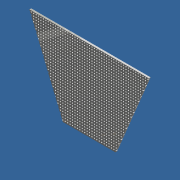
# Autodesk Inventor part: Detektorplatine
Saved by Autodesk Inventor 2018 (Build 220112000, 112)
## iProperties
Created: 2018-11-01
Part Number: Detektorplatine
Material: PC/ABS-Kunststoff
Document SubType Name: Modeling
Designer: M.Knabel
Density: 0.357273 g/cm^3
Appearance: Glatt - weiß
Mass: 2.14367 g
Surface Area: 141.537 cm^2
Volume: 6.0001 cm^3
Author: M.Knabel
Autodesk Inventor part; units mm, degrees
ref_plane "YZ Plane" through (0, 0, 0) normal (1, 0, 0) x (0, 1, 0)
ref_plane "XZ Plane" through (0, 0, 0) normal (0, 1, 0) x (-1, 0, 0)
ref_plane "XY Plane" through (0, 0, 0) normal (0, 0, 1) x (1, 0, 0)
sketch "Skizze1" plane through (0, 0, 0) normal (0, 1, 0) x (-1, 0, 0)
  line L0 (-50.2277, 69) -> (50.2277, 69)
  line L1 (50.2277, 69) -> (21.647, 0)
  line L2 (21.647, 0) -> (-21.647, 0)
  line L3 (-21.647, 0) -> (-50.2277, 69)
  line L4 (0, -13.8) -> (0, 82.8) construction
  line L5 (70.3188, 0) -> (-70.3188, 0) construction
  point P0 (0, 0)
  dimension "d0" = 43.294
  dimension "d1" = 112.5
  dimension "d2" = 69
  constraints: 8 end point, 1 collinear, 1 horizontal, 1 parallel, 1 other
  measures "d0" distance of L1.end L2.end
  measures "d1" angle of L2 L3
  measures "d2" distance between parallel lines of L2 L0
extrude "Extrusion1" add sketch "Skizze1" along normal blind 1.5
sketch "Skizze2" plane through (0, 1.5, 0) normal (0, 1, 0) x (1, 0, 0)
  line L0 (21.647, 0) -> (-21.647, 0) projected
  line L1 (-21.647, 0) -> (-21.647, 7.3765) construction
  point P0 (0, 0)
  point P1 (-21.647, -1.5)
  point P2 (-19.647, -1.5)
  point P3 (-17.647, -1.5)
  point P4 (-15.647, -1.5)
  point P5 (-13.647, -1.5)
  point P6 (-11.647, -1.5)
  point P7 (-9.647, -1.5)
  point P8 (-7.647, -1.5)
  point P9 (-5.647, -1.5)
  point P10 (-3.647, -1.5)
  point P11 (-1.647, -1.5)
  point P12 (0.353, -1.5)
  point P13 (2.353, -1.5)
  point P14 (4.353, -1.5)
  point P15 (6.353, -1.5)
  point P16 (8.353, -1.5)
  point P17 (10.353, -1.5)
  point P18 (12.353, -1.5)
  point P19 (14.353, -1.5)
  point P20 (16.353, -1.5)
  point P21 (18.353, -1.5)
  point P22 (20.353, -1.5)
  point P23 (22.353, -1.5)
  point P24 (22.353, -3.5)
  point P25 (20.353, -3.5)
  point P26 (18.353, -3.5)
  point P27 (16.353, -3.5)
  point P28 (14.353, -3.5)
  point P29 (12.353, -3.5)
  point P30 (10.353, -3.5)
  point P31 (8.353, -3.5)
  point P32 (6.353, -3.5)
  point P33 (4.353, -3.5)
  point P34 (2.353, -3.5)
  point P35 (0.353, -3.5)
  point P36 (-1.647, -3.5)
  point P37 (-3.647, -3.5)
  point P38 (-5.647, -3.5)
  point P39 (-7.647, -3.5)
  point P40 (-9.647, -3.5)
  point P41 (-11.647, -3.5)
  point P42 (-13.647, -3.5)
  point P43 (-15.647, -3.5)
  point P44 (-17.647, -3.5)
  point P45 (-19.647, -3.5)
  point P46 (-21.647, -3.5)
  point P47 (22.353, -5.5)
  point P48 (20.353, -5.5)
  point P49 (18.353, -5.5)
  point P50 (16.353, -5.5)
  point P51 (14.353, -5.5)
  point P52 (12.353, -5.5)
  point P53 (10.353, -5.5)
  point P54 (8.353, -5.5)
  point P55 (6.353, -5.5)
  point P56 (4.353, -5.5)
  point P57 (2.353, -5.5)
  point P58 (0.353, -5.5)
  point P59 (-1.647, -5.5)
  point P60 (-3.647, -5.5)
  point P61 (-5.647, -5.5)
  point P62 (-7.647, -5.5)
  point P63 (-9.647, -5.5)
  point P64 (-11.647, -5.5)
  point P65 (-13.647, -5.5)
  point P66 (-15.647, -5.5)
  point P67 (-17.647, -5.5)
  point P68 (-19.647, -5.5)
  point P69 (-21.647, -5.5)
  point P70 (22.353, -7.5)
  point P71 (20.353, -7.5)
  point P72 (18.353, -7.5)
  point P73 (16.353, -7.5)
  point P74 (14.353, -7.5)
  point P75 (12.353, -7.5)
  point P76 (10.353, -7.5)
  point P77 (8.353, -7.5)
  point P78 (6.353, -7.5)
  point P79 (4.353, -7.5)
  point P80 (2.353, -7.5)
  point P81 (0.353, -7.5)
  point P82 (-1.647, -7.5)
  point P83 (-3.647, -7.5)
  point P84 (-5.647, -7.5)
  point P85 (-7.647, -7.5)
  point P86 (-9.647, -7.5)
  point P87 (-11.647, -7.5)
  point P88 (-13.647, -7.5)
  point P89 (-15.647, -7.5)
  point P90 (-17.647, -7.5)
  point P91 (-19.647, -7.5)
  point P92 (-21.647, -7.5)
  point P93 (22.353, -9.5)
  point P94 (20.353, -9.5)
  point P95 (18.353, -9.5)
  point P96 (16.353, -9.5)
  point P97 (14.353, -9.5)
  point P98 (12.353, -9.5)
  point P99 (10.353, -9.5)
  point P100 (8.353, -9.5)
  point P101 (6.353, -9.5)
  point P102 (4.353, -9.5)
  point P103 (2.353, -9.5)
  point P104 (0.353, -9.5)
  point P105 (-1.647, -9.5)
  point P106 (-3.647, -9.5)
  point P107 (-5.647, -9.5)
  point P108 (-7.647, -9.5)
  point P109 (-9.647, -9.5)
  point P110 (-11.647, -9.5)
  point P111 (-13.647, -9.5)
  point P112 (-15.647, -9.5)
  point P113 (-17.647, -9.5)
  point P114 (-19.647, -9.5)
  point P115 (-21.647, -9.5)
  point P116 (22.353, -11.5)
  point P117 (20.353, -11.5)
  point P118 (18.353, -11.5)
  point P119 (16.353, -11.5)
  point P120 (14.353, -11.5)
  point P121 (12.353, -11.5)
  point P122 (10.353, -11.5)
  point P123 (8.353, -11.5)
  point P124 (6.353, -11.5)
  point P125 (4.353, -11.5)
  point P126 (2.353, -11.5)
  point P127 (0.353, -11.5)
  point P128 (-1.647, -11.5)
  point P129 (-3.647, -11.5)
  point P130 (-5.647, -11.5)
  point P131 (-7.647, -11.5)
  point P132 (-9.647, -11.5)
  point P133 (-11.647, -11.5)
  point P134 (-13.647, -11.5)
  point P135 (-15.647, -11.5)
  point P136 (-17.647, -11.5)
  point P137 (-19.647, -11.5)
  point P138 (-21.647, -11.5)
  point P139 (22.353, -13.5)
  point P140 (20.353, -13.5)
  point P141 (18.353, -13.5)
  point P142 (16.353, -13.5)
  point P143 (14.353, -13.5)
  point P144 (12.353, -13.5)
  point P145 (10.353, -13.5)
  point P146 (8.353, -13.5)
  point P147 (6.353, -13.5)
  point P148 (4.353, -13.5)
  point P149 (2.353, -13.5)
  point P150 (0.353, -13.5)
  point P151 (-1.647, -13.5)
  point P152 (-3.647, -13.5)
  point P153 (-5.647, -13.5)
  point P154 (-7.647, -13.5)
  point P155 (-9.647, -13.5)
  point P156 (-11.647, -13.5)
  point P157 (-13.647, -13.5)
  point P158 (-15.647, -13.5)
  point P159 (-17.647, -13.5)
  point P160 (-19.647, -13.5)
  point P161 (-21.647, -13.5)
  point P162 (22.353, -15.5)
  point P163 (20.353, -15.5)
  point P164 (18.353, -15.5)
  point P165 (16.353, -15.5)
  point P166 (14.353, -15.5)
  point P167 (12.353, -15.5)
  point P168 (10.353, -15.5)
  point P169 (8.353, -15.5)
  point P170 (6.353, -15.5)
  point P171 (4.353, -15.5)
  point P172 (2.353, -15.5)
  point P173 (0.353, -15.5)
  point P174 (-1.647, -15.5)
  point P175 (-3.647, -15.5)
  point P176 (-5.647, -15.5)
  point P177 (-7.647, -15.5)
  point P178 (-9.647, -15.5)
  point P179 (-11.647, -15.5)
  point P180 (-13.647, -15.5)
  point P181 (-15.647, -15.5)
  point P182 (-17.647, -15.5)
  point P183 (-19.647, -15.5)
  point P184 (-21.647, -15.5)
  point P185 (22.353, -17.5)
  point P186 (20.353, -17.5)
  point P187 (18.353, -17.5)
  point P188 (16.353, -17.5)
  point P189 (14.353, -17.5)
  point P190 (12.353, -17.5)
  point P191 (10.353, -17.5)
  point P192 (8.353, -17.5)
  point P193 (6.353, -17.5)
  point P194 (4.353, -17.5)
  point P195 (2.353, -17.5)
  point P196 (0.353, -17.5)
  point P197 (-1.647, -17.5)
  point P198 (-3.647, -17.5)
  point P199 (-5.647, -17.5)
  dimension "d5" = 1.5
  dimension "d8" = 2
  dimension "d15" = 2
  dimension "d22" = 2
  dimension "d29" = 2
  constraints: 3 horizontal, 2 end point, 2 vertical, 1 point on line, 1665 other
  measures "d5" distance from line of L0 point (-21.647, -1.5)
  measures "d8" distance of point (-21.647, -1.5) point (-19.647, -1.5)
  measures "d15" distance of point (22.353, -1.5) point (22.353, -3.5)
  measures "d22" distance of point (22.353, -67.5) point (24.353, -67.5)
  measures "d29" distance of point (-21.647, -67.5) point (-23.647, -67.5)
hole "Bohrung1" at (-21.647, 1.5, 1.5) at (-19.647, 1.5, 1.5) at (-17.647, 1.5, 1.5) at (-15.647, 1.5, 1.5) at (-13.647, 1.5, 1.5) at (-11.647, 1.5, 1.5) at (-9.647, 1.5, 1.5) at (-7.647, 1.5, 1.5) at (-5.647, 1.5, 1.5) at (-3.647, 1.5, 1.5) at (-1.647, 1.5, 1.5) at (0.353, 1.5, 1.5) at (2.353, 1.5, 1.5) at (4.353, 1.5, 1.5) at (6.353, 1.5, 1.5) at (8.353, 1.5, 1.5) at (10.353, 1.5, 1.5) at (12.353, 1.5, 1.5) at (14.353, 1.5, 1.5) at (16.353, 1.5, 1.5) at (18.353, 1.5, 1.5) at (20.353, 1.5, 1.5) at (22.353, 1.5, 1.5) at (22.353, 1.5, 3.5) at (20.353, 1.5, 3.5) at (18.353, 1.5, 3.5) at (16.353, 1.5, 3.5) at (14.353, 1.5, 3.5) at (12.353, 1.5, 3.5) at (10.353, 1.5, 3.5) at (8.353, 1.5, 3.5) at (6.353, 1.5, 3.5) at (4.353, 1.5, 3.5) at (2.353, 1.5, 3.5) at (0.353, 1.5, 3.5) at (-1.647, 1.5, 3.5) at (-3.647, 1.5, 3.5) at (-5.647, 1.5, 3.5) at (-7.647, 1.5, 3.5) at (-9.647, 1.5, 3.5) at (-11.647, 1.5, 3.5) at (-13.647, 1.5, 3.5) at (-15.647, 1.5, 3.5) at (-17.647, 1.5, 3.5) at (-19.647, 1.5, 3.5) at (-21.647, 1.5, 3.5) at (22.353, 1.5, 5.5) at (20.353, 1.5, 5.5) at (18.353, 1.5, 5.5) at (16.353, 1.5, 5.5) direction (0, -1, 0) diameter 1 end through all and at (14.353, 1.5, 5.5) (12.353, 1.5, 5.5) (10.353, 1.5, 5.5) (8.353, 1.5, 5.5) (6.353, 1.5, 5.5) (4.353, 1.5, 5.5) (2.353, 1.5, 5.5) (0.353, 1.5, 5.5) (-1.647, 1.5, 5.5) (-3.647, 1.5, 5.5) (-5.647, 1.5, 5.5) (-7.647, 1.5, 5.5) (-9.647, 1.5, 5.5) (-11.647, 1.5, 5.5) (-13.647, 1.5, 5.5) (-15.647, 1.5, 5.5) (-17.647, 1.5, 5.5) (-19.647, 1.5, 5.5) (-21.647, 1.5, 5.5) (22.353, 1.5, 7.5) (20.353, 1.5, 7.5) (18.353, 1.5, 7.5) (16.353, 1.5, 7.5) (14.353, 1.5, 7.5) (12.353, 1.5, 7.5) (10.353, 1.5, 7.5) (8.353, 1.5, 7.5) (6.353, 1.5, 7.5) (4.353, 1.5, 7.5) (2.353, 1.5, 7.5) (0.353, 1.5, 7.5) (-1.647, 1.5, 7.5) (-3.647, 1.5, 7.5) (-5.647, 1.5, 7.5) (-7.647, 1.5, 7.5) (-9.647, 1.5, 7.5) (-11.647, 1.5, 7.5) (-13.647, 1.5, 7.5) (-15.647, 1.5, 7.5) (-17.647, 1.5, 7.5) (-19.647, 1.5, 7.5) (-21.647, 1.5, 7.5) (22.353, 1.5, 9.5) (20.353, 1.5, 9.5) (18.353, 1.5, 9.5) (16.353, 1.5, 9.5) (14.353, 1.5, 9.5) (12.353, 1.5, 9.5) (10.353, 1.5, 9.5) (8.353, 1.5, 9.5) (6.353, 1.5, 9.5) (4.353, 1.5, 9.5) (2.353, 1.5, 9.5) (0.353, 1.5, 9.5) (-1.647, 1.5, 9.5) (-3.647, 1.5, 9.5) (-5.647, 1.5, 9.5) (-7.647, 1.5, 9.5) (-9.647, 1.5, 9.5) (-11.647, 1.5, 9.5) (-13.647, 1.5, 9.5) (-15.647, 1.5, 9.5) (-17.647, 1.5, 9.5) (-19.647, 1.5, 9.5) (-21.647, 1.5, 9.5) (22.353, 1.5, 11.5) (20.353, 1.5, 11.5) (18.353, 1.5, 11.5) (16.353, 1.5, 11.5) (14.353, 1.5, 11.5) (12.353, 1.5, 11.5) (10.353, 1.5, 11.5) (8.353, 1.5, 11.5) (6.353, 1.5, 11.5) (4.353, 1.5, 11.5) (2.353, 1.5, 11.5) (0.353, 1.5, 11.5) (-1.647, 1.5, 11.5) (-3.647, 1.5, 11.5) (-5.647, 1.5, 11.5) (-7.647, 1.5, 11.5) (-9.647, 1.5, 11.5) (-11.647, 1.5, 11.5) (-13.647, 1.5, 11.5) (-15.647, 1.5, 11.5) (-17.647, 1.5, 11.5) (-19.647, 1.5, 11.5) (-21.647, 1.5, 11.5) (22.353, 1.5, 13.5) (20.353, 1.5, 13.5) (18.353, 1.5, 13.5) (16.353, 1.5, 13.5) (14.353, 1.5, 13.5) (12.353, 1.5, 13.5) (10.353, 1.5, 13.5) (8.353, 1.5, 13.5) (6.353, 1.5, 13.5) (4.353, 1.5, 13.5) (2.353, 1.5, 13.5) (0.353, 1.5, 13.5) (-1.647, 1.5, 13.5) (-3.647, 1.5, 13.5) (-5.647, 1.5, 13.5) (-7.647, 1.5, 13.5) (-9.647, 1.5, 13.5) (-11.647, 1.5, 13.5) (-13.647, 1.5, 13.5) (-15.647, 1.5, 13.5) (-17.647, 1.5, 13.5) (-19.647, 1.5, 13.5) (-21.647, 1.5, 13.5) (22.353, 1.5, 15.5) (20.353, 1.5, 15.5) (18.353, 1.5, 15.5) (16.353, 1.5, 15.5) (14.353, 1.5, 15.5) (12.353, 1.5, 15.5) (10.353, 1.5, 15.5) (8.353, 1.5, 15.5) (6.353, 1.5, 15.5) (4.353, 1.5, 15.5) (2.353, 1.5, 15.5) (0.353, 1.5, 15.5) (-1.647, 1.5, 15.5) (-3.647, 1.5, 15.5) (-5.647, 1.5, 15.5) (-7.647, 1.5, 15.5) (-9.647, 1.5, 15.5) (-11.647, 1.5, 15.5) (-13.647, 1.5, 15.5) (-15.647, 1.5, 15.5) (-17.647, 1.5, 15.5) (-19.647, 1.5, 15.5) (-21.647, 1.5, 15.5) (22.353, 1.5, 17.5) (20.353, 1.5, 17.5) (18.353, 1.5, 17.5) (16.353, 1.5, 17.5) (14.353, 1.5, 17.5) (12.353, 1.5, 17.5) (10.353, 1.5, 17.5) (8.353, 1.5, 17.5) (6.353, 1.5, 17.5) (4.353, 1.5, 17.5) (2.353, 1.5, 17.5) (0.353, 1.5, 17.5) (-1.647, 1.5, 17.5) (-3.647, 1.5, 17.5) (-5.647, 1.5, 17.5) (-7.647, 1.5, 17.5) (-9.647, 1.5, 17.5) (-11.647, 1.5, 17.5) (-13.647, 1.5, 17.5) (-15.647, 1.5, 17.5) (-17.647, 1.5, 17.5) (-19.647, 1.5, 17.5) (-21.647, 1.5, 17.5) (22.353, 1.5, 19.5) (20.353, 1.5, 19.5) (18.353, 1.5, 19.5) (16.353, 1.5, 19.5) (14.353, 1.5, 19.5) (12.353, 1.5, 19.5) (10.353, 1.5, 19.5) (8.353, 1.5, 19.5) (6.353, 1.5, 19.5) (4.353, 1.5, 19.5) (2.353, 1.5, 19.5) (0.353, 1.5, 19.5) (-1.647, 1.5, 19.5) (-3.647, 1.5, 19.5) (-5.647, 1.5, 19.5) (-7.647, 1.5, 19.5) (-9.647, 1.5, 19.5) (-11.647, 1.5, 19.5) (-13.647, 1.5, 19.5) (-15.647, 1.5, 19.5) (-17.647, 1.5, 19.5) (-19.647, 1.5, 19.5) (-21.647, 1.5, 19.5) (22.353, 1.5, 21.5) (20.353, 1.5, 21.5) (18.353, 1.5, 21.5) (16.353, 1.5, 21.5) (14.353, 1.5, 21.5) (12.353, 1.5, 21.5) (10.353, 1.5, 21.5) (8.353, 1.5, 21.5) (6.353, 1.5, 21.5) (4.353, 1.5, 21.5) (2.353, 1.5, 21.5) (0.353, 1.5, 21.5) (-1.647, 1.5, 21.5) (-3.647, 1.5, 21.5) (-5.647, 1.5, 21.5) (-7.647, 1.5, 21.5) (-9.647, 1.5, 21.5) (-11.647, 1.5, 21.5) (-13.647, 1.5, 21.5) (-15.647, 1.5, 21.5) (-17.647, 1.5, 21.5) (-19.647, 1.5, 21.5) (-21.647, 1.5, 21.5) (22.353, 1.5, 23.5) (20.353, 1.5, 23.5) (18.353, 1.5, 23.5) (16.353, 1.5, 23.5) (14.353, 1.5, 23.5) (12.353, 1.5, 23.5) (10.353, 1.5, 23.5) (8.353, 1.5, 23.5) (6.353, 1.5, 23.5) (4.353, 1.5, 23.5) (2.353, 1.5, 23.5) (0.353, 1.5, 23.5) (-1.647, 1.5, 23.5) (-3.647, 1.5, 23.5) (-5.647, 1.5, 23.5) (-7.647, 1.5, 23.5) (-9.647, 1.5, 23.5) (-11.647, 1.5, 23.5) (-13.647, 1.5, 23.5) (-15.647, 1.5, 23.5) (-17.647, 1.5, 23.5) (-19.647, 1.5, 23.5) (-21.647, 1.5, 23.5) (22.353, 1.5, 25.5) (20.353, 1.5, 25.5) (18.353, 1.5, 25.5) (16.353, 1.5, 25.5) (14.353, 1.5, 25.5) (12.353, 1.5, 25.5) (10.353, 1.5, 25.5) (8.353, 1.5, 25.5) (6.353, 1.5, 25.5) (4.353, 1.5, 25.5) (2.353, 1.5, 25.5) (0.353, 1.5, 25.5) (-1.647, 1.5, 25.5) (-3.647, 1.5, 25.5) (-5.647, 1.5, 25.5) (-7.647, 1.5, 25.5) (-9.647, 1.5, 25.5) (-11.647, 1.5, 25.5) (-13.647, 1.5, 25.5) (-15.647, 1.5, 25.5) (-17.647, 1.5, 25.5) (-19.647, 1.5, 25.5) (-21.647, 1.5, 25.5) (22.353, 1.5, 27.5) (20.353, 1.5, 27.5) (18.353, 1.5, 27.5) (16.353, 1.5, 27.5) (14.353, 1.5, 27.5) (12.353, 1.5, 27.5) (10.353, 1.5, 27.5) (8.353, 1.5, 27.5) (6.353, 1.5, 27.5) (4.353, 1.5, 27.5) (2.353, 1.5, 27.5) (0.353, 1.5, 27.5) (-1.647, 1.5, 27.5) (-3.647, 1.5, 27.5) (-5.647, 1.5, 27.5) (-7.647, 1.5, 27.5) (-9.647, 1.5, 27.5) (-11.647, 1.5, 27.5) (-13.647, 1.5, 27.5) (-15.647, 1.5, 27.5) (-17.647, 1.5, 27.5) (-19.647, 1.5, 27.5) (-21.647, 1.5, 27.5) (22.353, 1.5, 29.5) (20.353, 1.5, 29.5) (18.353, 1.5, 29.5) (16.353, 1.5, 29.5) (14.353, 1.5, 29.5) (12.353, 1.5, 29.5) (10.353, 1.5, 29.5) (8.353, 1.5, 29.5) (6.353, 1.5, 29.5) (4.353, 1.5, 29.5) (2.353, 1.5, 29.5) (0.353, 1.5, 29.5) (-1.647, 1.5, 29.5) (-3.647, 1.5, 29.5) (-5.647, 1.5, 29.5) (-7.647, 1.5, 29.5) (-9.647, 1.5, 29.5) (-11.647, 1.5, 29.5) (-13.647, 1.5, 29.5) (-15.647, 1.5, 29.5) (-17.647, 1.5, 29.5) (-19.647, 1.5, 29.5) (-21.647, 1.5, 29.5) (22.353, 1.5, 31.5) (20.353, 1.5, 31.5) (18.353, 1.5, 31.5) (16.353, 1.5, 31.5) (14.353, 1.5, 31.5) (12.353, 1.5, 31.5) (10.353, 1.5, 31.5) (8.353, 1.5, 31.5) (6.353, 1.5, 31.5) (4.353, 1.5, 31.5) (2.353, 1.5, 31.5) (0.353, 1.5, 31.5) (-1.647, 1.5, 31.5) (-3.647, 1.5, 31.5) (-5.647, 1.5, 31.5) (-7.647, 1.5, 31.5) (-9.647, 1.5, 31.5) (-11.647, 1.5, 31.5) (-13.647, 1.5, 31.5) (-15.647, 1.5, 31.5) (-17.647, 1.5, 31.5) (-19.647, 1.5, 31.5) (-21.647, 1.5, 31.5) (22.353, 1.5, 33.5) (20.353, 1.5, 33.5) (18.353, 1.5, 33.5) (16.353, 1.5, 33.5) (14.353, 1.5, 33.5) (12.353, 1.5, 33.5) (10.353, 1.5, 33.5) (8.353, 1.5, 33.5) (6.353, 1.5, 33.5) (4.353, 1.5, 33.5) (2.353, 1.5, 33.5) (0.353, 1.5, 33.5) (-1.647, 1.5, 33.5) (-3.647, 1.5, 33.5) (-5.647, 1.5, 33.5) (-7.647, 1.5, 33.5) (-9.647, 1.5, 33.5) (-11.647, 1.5, 33.5) (-13.647, 1.5, 33.5) (-15.647, 1.5, 33.5) (-17.647, 1.5, 33.5) (-19.647, 1.5, 33.5) (-21.647, 1.5, 33.5) (22.353, 1.5, 35.5) (20.353, 1.5, 35.5) (18.353, 1.5, 35.5) (16.353, 1.5, 35.5) (14.353, 1.5, 35.5) (12.353, 1.5, 35.5) (10.353, 1.5, 35.5) (8.353, 1.5, 35.5) (6.353, 1.5, 35.5) (4.353, 1.5, 35.5) (2.353, 1.5, 35.5) (0.353, 1.5, 35.5) (-1.647, 1.5, 35.5) (-3.647, 1.5, 35.5) (-5.647, 1.5, 35.5) (-7.647, 1.5, 35.5) (-9.647, 1.5, 35.5) (-11.647, 1.5, 35.5) (-13.647, 1.5, 35.5) (-15.647, 1.5, 35.5) (-17.647, 1.5, 35.5) (-19.647, 1.5, 35.5) (-21.647, 1.5, 35.5) (22.353, 1.5, 37.5) (20.353, 1.5, 37.5) (18.353, 1.5, 37.5) (16.353, 1.5, 37.5) (14.353, 1.5, 37.5) (12.353, 1.5, 37.5) (10.353, 1.5, 37.5) (8.353, 1.5, 37.5) (6.353, 1.5, 37.5) (4.353, 1.5, 37.5) (2.353, 1.5, 37.5) (0.353, 1.5, 37.5) (-1.647, 1.5, 37.5) (-3.647, 1.5, 37.5) (-5.647, 1.5, 37.5) (-7.647, 1.5, 37.5) (-9.647, 1.5, 37.5) (-11.647, 1.5, 37.5) (-13.647, 1.5, 37.5) (-15.647, 1.5, 37.5) (-17.647, 1.5, 37.5) (-19.647, 1.5, 37.5) (-21.647, 1.5, 37.5) (22.353, 1.5, 39.5) (20.353, 1.5, 39.5) (18.353, 1.5, 39.5) (16.353, 1.5, 39.5) (14.353, 1.5, 39.5) (12.353, 1.5, 39.5) (10.353, 1.5, 39.5) (8.353, 1.5, 39.5) (6.353, 1.5, 39.5) (4.353, 1.5, 39.5) (2.353, 1.5, 39.5) (0.353, 1.5, 39.5) (-1.647, 1.5, 39.5) (-3.647, 1.5, 39.5) (-5.647, 1.5, 39.5) (-7.647, 1.5, 39.5) (-9.647, 1.5, 39.5) (-11.647, 1.5, 39.5) (-13.647, 1.5, 39.5) (-15.647, 1.5, 39.5) (-17.647, 1.5, 39.5) (-19.647, 1.5, 39.5) (-21.647, 1.5, 39.5) (22.353, 1.5, 41.5) (20.353, 1.5, 41.5) (18.353, 1.5, 41.5) (16.353, 1.5, 41.5) (14.353, 1.5, 41.5) (12.353, 1.5, 41.5) (10.353, 1.5, 41.5) (8.353, 1.5, 41.5) (6.353, 1.5, 41.5) (4.353, 1.5, 41.5) (2.353, 1.5, 41.5) (0.353, 1.5, 41.5) (-1.647, 1.5, 41.5) (-3.647, 1.5, 41.5) (-5.647, 1.5, 41.5) (-7.647, 1.5, 41.5) (-9.647, 1.5, 41.5) (-11.647, 1.5, 41.5) (-13.647, 1.5, 41.5) (-15.647, 1.5, 41.5) (-17.647, 1.5, 41.5) (-19.647, 1.5, 41.5) (-21.647, 1.5, 41.5) (22.353, 1.5, 43.5) (20.353, 1.5, 43.5) (18.353, 1.5, 43.5) (16.353, 1.5, 43.5) (14.353, 1.5, 43.5) (12.353, 1.5, 43.5) (10.353, 1.5, 43.5) (8.353, 1.5, 43.5) (6.353, 1.5, 43.5) (4.353, 1.5, 43.5) (2.353, 1.5, 43.5) (0.353, 1.5, 43.5) (-1.647, 1.5, 43.5) (-3.647, 1.5, 43.5) (-5.647, 1.5, 43.5) (-7.647, 1.5, 43.5) (-9.647, 1.5, 43.5) (-11.647, 1.5, 43.5) (-13.647, 1.5, 43.5) (-15.647, 1.5, 43.5) (-17.647, 1.5, 43.5) (-19.647, 1.5, 43.5) (-21.647, 1.5, 43.5) (22.353, 1.5, 45.5) (20.353, 1.5, 45.5) (18.353, 1.5, 45.5) (16.353, 1.5, 45.5) (14.353, 1.5, 45.5) (12.353, 1.5, 45.5) (10.353, 1.5, 45.5) (8.353, 1.5, 45.5) (6.353, 1.5, 45.5) (4.353, 1.5, 45.5) (2.353, 1.5, 45.5) (0.353, 1.5, 45.5) (-1.647, 1.5, 45.5) (-3.647, 1.5, 45.5) (-5.647, 1.5, 45.5) (-7.647, 1.5, 45.5) (-9.647, 1.5, 45.5) (-11.647, 1.5, 45.5) (-13.647, 1.5, 45.5) (-15.647, 1.5, 45.5) (-17.647, 1.5, 45.5) (-19.647, 1.5, 45.5) (-21.647, 1.5, 45.5) (22.353, 1.5, 47.5) (20.353, 1.5, 47.5) (18.353, 1.5, 47.5) (16.353, 1.5, 47.5) (14.353, 1.5, 47.5) (12.353, 1.5, 47.5) (10.353, 1.5, 47.5) (8.353, 1.5, 47.5) (6.353, 1.5, 47.5) (4.353, 1.5, 47.5) (2.353, 1.5, 47.5) (0.353, 1.5, 47.5) (-1.647, 1.5, 47.5) (-3.647, 1.5, 47.5) (-5.647, 1.5, 47.5) (-7.647, 1.5, 47.5) (-9.647, 1.5, 47.5) (-11.647, 1.5, 47.5) (-13.647, 1.5, 47.5) (-15.647, 1.5, 47.5) (-17.647, 1.5, 47.5) (-19.647, 1.5, 47.5) (-21.647, 1.5, 47.5) (22.353, 1.5, 49.5) (20.353, 1.5, 49.5) (18.353, 1.5, 49.5) (16.353, 1.5, 49.5) (14.353, 1.5, 49.5) (12.353, 1.5, 49.5) (10.353, 1.5, 49.5) (8.353, 1.5, 49.5) (6.353, 1.5, 49.5) (4.353, 1.5, 49.5) (2.353, 1.5, 49.5) (0.353, 1.5, 49.5) (-1.647, 1.5, 49.5) (-3.647, 1.5, 49.5) (-5.647, 1.5, 49.5) (-7.647, 1.5, 49.5) (-9.647, 1.5, 49.5) (-11.647, 1.5, 49.5) (-13.647, 1.5, 49.5) (-15.647, 1.5, 49.5) (-17.647, 1.5, 49.5) (-19.647, 1.5, 49.5) (-21.647, 1.5, 49.5) (22.353, 1.5, 51.5) (20.353, 1.5, 51.5) (18.353, 1.5, 51.5) (16.353, 1.5, 51.5) (14.353, 1.5, 51.5) (12.353, 1.5, 51.5) (10.353, 1.5, 51.5) (8.353, 1.5, 51.5) (6.353, 1.5, 51.5) (4.353, 1.5, 51.5) (2.353, 1.5, 51.5) (0.353, 1.5, 51.5) (-1.647, 1.5, 51.5) (-3.647, 1.5, 51.5) (-5.647, 1.5, 51.5) (-7.647, 1.5, 51.5) (-9.647, 1.5, 51.5) (-11.647, 1.5, 51.5) (-13.647, 1.5, 51.5) (-15.647, 1.5, 51.5) (-17.647, 1.5, 51.5) (-19.647, 1.5, 51.5) (-21.647, 1.5, 51.5) (22.353, 1.5, 53.5) (20.353, 1.5, 53.5) (18.353, 1.5, 53.5) (16.353, 1.5, 53.5) (14.353, 1.5, 53.5) (12.353, 1.5, 53.5) (10.353, 1.5, 53.5) (8.353, 1.5, 53.5) (6.353, 1.5, 53.5) (4.353, 1.5, 53.5) (2.353, 1.5, 53.5) (0.353, 1.5, 53.5) (-1.647, 1.5, 53.5) (-3.647, 1.5, 53.5) (-5.647, 1.5, 53.5) (-7.647, 1.5, 53.5) (-9.647, 1.5, 53.5) (-11.647, 1.5, 53.5) (-13.647, 1.5, 53.5) (-15.647, 1.5, 53.5) (-17.647, 1.5, 53.5) (-19.647, 1.5, 53.5) (-21.647, 1.5, 53.5) (22.353, 1.5, 55.5) (20.353, 1.5, 55.5) (18.353, 1.5, 55.5) (16.353, 1.5, 55.5) (14.353, 1.5, 55.5) (12.353, 1.5, 55.5) (10.353, 1.5, 55.5) (8.353, 1.5, 55.5) (6.353, 1.5, 55.5) (4.353, 1.5, 55.5) (2.353, 1.5, 55.5) (0.353, 1.5, 55.5) (-1.647, 1.5, 55.5) (-3.647, 1.5, 55.5) (-5.647, 1.5, 55.5) (-7.647, 1.5, 55.5) (-9.647, 1.5, 55.5) (-11.647, 1.5, 55.5) (-13.647, 1.5, 55.5) (-15.647, 1.5, 55.5) (-17.647, 1.5, 55.5) (-19.647, 1.5, 55.5) (-21.647, 1.5, 55.5) (22.353, 1.5, 57.5) (20.353, 1.5, 57.5) (18.353, 1.5, 57.5) (16.353, 1.5, 57.5) (14.353, 1.5, 57.5) (12.353, 1.5, 57.5) (10.353, 1.5, 57.5) (8.353, 1.5, 57.5) (6.353, 1.5, 57.5) (4.353, 1.5, 57.5) (2.353, 1.5, 57.5) (0.353, 1.5, 57.5) (-1.647, 1.5, 57.5) (-3.647, 1.5, 57.5) (-5.647, 1.5, 57.5) (-7.647, 1.5, 57.5) (-9.647, 1.5, 57.5) (-11.647, 1.5, 57.5) (-13.647, 1.5, 57.5) (-15.647, 1.5, 57.5) (-17.647, 1.5, 57.5) (-19.647, 1.5, 57.5) (-21.647, 1.5, 57.5) (22.353, 1.5, 59.5) (20.353, 1.5, 59.5) (18.353, 1.5, 59.5) (16.353, 1.5, 59.5) (14.353, 1.5, 59.5) (12.353, 1.5, 59.5) (10.353, 1.5, 59.5) (8.353, 1.5, 59.5) (6.353, 1.5, 59.5) (4.353, 1.5, 59.5) (2.353, 1.5, 59.5) (0.353, 1.5, 59.5) (-1.647, 1.5, 59.5) (-3.647, 1.5, 59.5) (-5.647, 1.5, 59.5) (-7.647, 1.5, 59.5) (-9.647, 1.5, 59.5) (-11.647, 1.5, 59.5) (-13.647, 1.5, 59.5) (-15.647, 1.5, 59.5) (-17.647, 1.5, 59.5) (-19.647, 1.5, 59.5) (-21.647, 1.5, 59.5) (22.353, 1.5, 61.5) (20.353, 1.5, 61.5) (18.353, 1.5, 61.5) (16.353, 1.5, 61.5) (14.353, 1.5, 61.5) (12.353, 1.5, 61.5) (10.353, 1.5, 61.5) (8.353, 1.5, 61.5) (6.353, 1.5, 61.5) (4.353, 1.5, 61.5) (2.353, 1.5, 61.5) (0.353, 1.5, 61.5) (-1.647, 1.5, 61.5) (-3.647, 1.5, 61.5) (-5.647, 1.5, 61.5) (-7.647, 1.5, 61.5) (-9.647, 1.5, 61.5) (-11.647, 1.5, 61.5) (-13.647, 1.5, 61.5) (-15.647, 1.5, 61.5) (-17.647, 1.5, 61.5) (-19.647, 1.5, 61.5) (-21.647, 1.5, 61.5) (22.353, 1.5, 63.5) (20.353, 1.5, 63.5) (18.353, 1.5, 63.5) (16.353, 1.5, 63.5) (14.353, 1.5, 63.5) (12.353, 1.5, 63.5) (10.353, 1.5, 63.5) (8.353, 1.5, 63.5) (6.353, 1.5, 63.5) (4.353, 1.5, 63.5) (2.353, 1.5, 63.5) (0.353, 1.5, 63.5) (-1.647, 1.5, 63.5) (-3.647, 1.5, 63.5) (-5.647, 1.5, 63.5) (-7.647, 1.5, 63.5) (-9.647, 1.5, 63.5) (-11.647, 1.5, 63.5) (-13.647, 1.5, 63.5) (-15.647, 1.5, 63.5) (-17.647, 1.5, 63.5) (-19.647, 1.5, 63.5) (-21.647, 1.5, 63.5) (22.353, 1.5, 65.5) (20.353, 1.5, 65.5) (18.353, 1.5, 65.5) (16.353, 1.5, 65.5) (14.353, 1.5, 65.5) (12.353, 1.5, 65.5) (10.353, 1.5, 65.5) (8.353, 1.5, 65.5) (6.353, 1.5, 65.5) (4.353, 1.5, 65.5) (2.353, 1.5, 65.5) (0.353, 1.5, 65.5) (-1.647, 1.5, 65.5) (-3.647, 1.5, 65.5) (-5.647, 1.5, 65.5) (-7.647, 1.5, 65.5) (-9.647, 1.5, 65.5) (-11.647, 1.5, 65.5) (-13.647, 1.5, 65.5) (-15.647, 1.5, 65.5) (-17.647, 1.5, 65.5) (-19.647, 1.5, 65.5) (-21.647, 1.5, 65.5) (22.353, 1.5, 67.5) (20.353, 1.5, 67.5) (18.353, 1.5, 67.5) (16.353, 1.5, 67.5) (14.353, 1.5, 67.5) (12.353, 1.5, 67.5) (10.353, 1.5, 67.5) (8.353, 1.5, 67.5) (6.353, 1.5, 67.5) (4.353, 1.5, 67.5) (2.353, 1.5, 67.5) (0.353, 1.5, 67.5) (-1.647, 1.5, 67.5) (-3.647, 1.5, 67.5) (-5.647, 1.5, 67.5) (-7.647, 1.5, 67.5) (-9.647, 1.5, 67.5) (-11.647, 1.5, 67.5) (-13.647, 1.5, 67.5) (-15.647, 1.5, 67.5) (-17.647, 1.5, 67.5) (-19.647, 1.5, 67.5) (-21.647, 1.5, 67.5) (24.353, 1.5, 67.5) (24.353, 1.5, 65.5) (24.353, 1.5, 63.5) (24.353, 1.5, 61.5) (24.353, 1.5, 59.5) (24.353, 1.5, 57.5) (24.353, 1.5, 55.5) (24.353, 1.5, 53.5) (24.353, 1.5, 51.5) (24.353, 1.5, 49.5) (24.353, 1.5, 47.5) (24.353, 1.5, 45.5) (24.353, 1.5, 43.5) (24.353, 1.5, 41.5) (24.353, 1.5, 39.5) (24.353, 1.5, 37.5) (24.353, 1.5, 35.5) (24.353, 1.5, 33.5) (24.353, 1.5, 31.5) (24.353, 1.5, 29.5) (24.353, 1.5, 27.5) (24.353, 1.5, 25.5) (24.353, 1.5, 23.5) (24.353, 1.5, 21.5) (24.353, 1.5, 19.5) (24.353, 1.5, 17.5) (24.353, 1.5, 15.5) (24.353, 1.5, 13.5) (24.353, 1.5, 11.5) (24.353, 1.5, 9.5) (24.353, 1.5, 7.5) (24.353, 1.5, 5.5) (24.353, 1.5, 3.5) (24.353, 1.5, 1.5) (26.353, 1.5, 67.5) (26.353, 1.5, 65.5) (26.353, 1.5, 63.5) (26.353, 1.5, 61.5) (26.353, 1.5, 59.5) (26.353, 1.5, 57.5) (26.353, 1.5, 55.5) (26.353, 1.5, 53.5) (26.353, 1.5, 51.5) (26.353, 1.5, 49.5) (26.353, 1.5, 47.5) (26.353, 1.5, 45.5) (26.353, 1.5, 43.5) (26.353, 1.5, 41.5) (26.353, 1.5, 39.5) (26.353, 1.5, 37.5) (26.353, 1.5, 35.5) (26.353, 1.5, 33.5) (26.353, 1.5, 31.5) (26.353, 1.5, 29.5) (26.353, 1.5, 27.5) (26.353, 1.5, 25.5) (26.353, 1.5, 23.5) (26.353, 1.5, 21.5) (26.353, 1.5, 19.5) (26.353, 1.5, 17.5) (26.353, 1.5, 15.5) (26.353, 1.5, 13.5) (26.353, 1.5, 11.5) (26.353, 1.5, 9.5) (26.353, 1.5, 7.5) (26.353, 1.5, 5.5) (26.353, 1.5, 3.5) (26.353, 1.5, 1.5) (28.353, 1.5, 67.5) (28.353, 1.5, 65.5) (28.353, 1.5, 63.5) (28.353, 1.5, 61.5) (28.353, 1.5, 59.5) (28.353, 1.5, 57.5) (28.353, 1.5, 55.5) (28.353, 1.5, 53.5) (28.353, 1.5, 51.5) (28.353, 1.5, 49.5) (28.353, 1.5, 47.5) (28.353, 1.5, 45.5) (28.353, 1.5, 43.5) (28.353, 1.5, 41.5) (28.353, 1.5, 39.5) (28.353, 1.5, 37.5) (28.353, 1.5, 35.5) (28.353, 1.5, 33.5) (28.353, 1.5, 31.5) (28.353, 1.5, 29.5) (28.353, 1.5, 27.5) (28.353, 1.5, 25.5) (28.353, 1.5, 23.5) (28.353, 1.5, 21.5) (28.353, 1.5, 19.5) (28.353, 1.5, 17.5) (28.353, 1.5, 15.5) (28.353, 1.5, 13.5) (28.353, 1.5, 11.5) (28.353, 1.5, 9.5) (28.353, 1.5, 7.5) (28.353, 1.5, 5.5) (28.353, 1.5, 3.5) (28.353, 1.5, 1.5) (30.353, 1.5, 67.5) (30.353, 1.5, 65.5) (30.353, 1.5, 63.5) (30.353, 1.5, 61.5) (30.353, 1.5, 59.5) (30.353, 1.5, 57.5) (30.353, 1.5, 55.5) (30.353, 1.5, 53.5) (30.353, 1.5, 51.5) (30.353, 1.5, 49.5) (30.353, 1.5, 47.5) (30.353, 1.5, 45.5) (30.353, 1.5, 43.5) (30.353, 1.5, 41.5) (30.353, 1.5, 39.5) (30.353, 1.5, 37.5) (30.353, 1.5, 35.5) (30.353, 1.5, 33.5) (30.353, 1.5, 31.5) (30.353, 1.5, 29.5) (30.353, 1.5, 27.5) (30.353, 1.5, 25.5) (30.353, 1.5, 23.5) (30.353, 1.5, 21.5) (30.353, 1.5, 19.5) (30.353, 1.5, 17.5) (30.353, 1.5, 15.5) (30.353, 1.5, 13.5) (30.353, 1.5, 11.5) (30.353, 1.5, 9.5) (30.353, 1.5, 7.5) (30.353, 1.5, 5.5) (30.353, 1.5, 3.5) (30.353, 1.5, 1.5) (32.353, 1.5, 67.5) (32.353, 1.5, 65.5) (32.353, 1.5, 63.5) (32.353, 1.5, 61.5) (32.353, 1.5, 59.5) (32.353, 1.5, 57.5) (32.353, 1.5, 55.5) (32.353, 1.5, 53.5) (32.353, 1.5, 51.5) (32.353, 1.5, 49.5) (32.353, 1.5, 47.5) (32.353, 1.5, 45.5) (32.353, 1.5, 43.5) (32.353, 1.5, 41.5) (32.353, 1.5, 39.5) (32.353, 1.5, 37.5) (32.353, 1.5, 35.5) (32.353, 1.5, 33.5) (32.353, 1.5, 31.5) (32.353, 1.5, 29.5) (32.353, 1.5, 27.5) (32.353, 1.5, 25.5) (32.353, 1.5, 23.5) (32.353, 1.5, 21.5) (32.353, 1.5, 19.5) (32.353, 1.5, 17.5) (32.353, 1.5, 15.5) (32.353, 1.5, 13.5) (32.353, 1.5, 11.5) (32.353, 1.5, 9.5) (32.353, 1.5, 7.5) (32.353, 1.5, 5.5) (32.353, 1.5, 3.5) (32.353, 1.5, 1.5) (34.353, 1.5, 67.5) (34.353, 1.5, 65.5) (34.353, 1.5, 63.5) (34.353, 1.5, 61.5) (34.353, 1.5, 59.5) (34.353, 1.5, 57.5) (34.353, 1.5, 55.5) (34.353, 1.5, 53.5) (34.353, 1.5, 51.5) (34.353, 1.5, 49.5) (34.353, 1.5, 47.5) (34.353, 1.5, 45.5) (34.353, 1.5, 43.5) (34.353, 1.5, 41.5) (34.353, 1.5, 39.5) (34.353, 1.5, 37.5) (34.353, 1.5, 35.5) (34.353, 1.5, 33.5) (34.353, 1.5, 31.5) (34.353, 1.5, 29.5) (34.353, 1.5, 27.5) (34.353, 1.5, 25.5) (34.353, 1.5, 23.5) (34.353, 1.5, 21.5) (34.353, 1.5, 19.5) (34.353, 1.5, 17.5) (34.353, 1.5, 15.5) (34.353, 1.5, 13.5) (34.353, 1.5, 11.5) (34.353, 1.5, 9.5) (34.353, 1.5, 7.5) (34.353, 1.5, 5.5) (34.353, 1.5, 3.5) (34.353, 1.5, 1.5) (36.353, 1.5, 67.5) (36.353, 1.5, 65.5) (36.353, 1.5, 63.5) (36.353, 1.5, 61.5) (36.353, 1.5, 59.5) (36.353, 1.5, 57.5) (36.353, 1.5, 55.5) (36.353, 1.5, 53.5) (36.353, 1.5, 51.5) (36.353, 1.5, 49.5) (36.353, 1.5, 47.5) (36.353, 1.5, 45.5) (36.353, 1.5, 43.5) (36.353, 1.5, 41.5) (36.353, 1.5, 39.5) (36.353, 1.5, 37.5) (36.353, 1.5, 35.5) (36.353, 1.5, 33.5) (36.353, 1.5, 31.5) (36.353, 1.5, 29.5) (36.353, 1.5, 27.5) (36.353, 1.5, 25.5) (36.353, 1.5, 23.5) (36.353, 1.5, 21.5) (36.353, 1.5, 19.5) (36.353, 1.5, 17.5) (36.353, 1.5, 15.5) (36.353, 1.5, 13.5) (36.353, 1.5, 11.5) (36.353, 1.5, 9.5) (36.353, 1.5, 7.5) (36.353, 1.5, 5.5) (36.353, 1.5, 3.5) (36.353, 1.5, 1.5) (38.353, 1.5, 67.5) (38.353, 1.5, 65.5) (38.353, 1.5, 63.5) (38.353, 1.5, 61.5) (38.353, 1.5, 59.5) (38.353, 1.5, 57.5) (38.353, 1.5, 55.5) (38.353, 1.5, 53.5) (38.353, 1.5, 51.5) (38.353, 1.5, 49.5) (38.353, 1.5, 47.5) (38.353, 1.5, 45.5) (38.353, 1.5, 43.5) (38.353, 1.5, 41.5) (38.353, 1.5, 39.5) (38.353, 1.5, 37.5) (38.353, 1.5, 35.5) (38.353, 1.5, 33.5) (38.353, 1.5, 31.5) (38.353, 1.5, 29.5) (38.353, 1.5, 27.5) (38.353, 1.5, 25.5) (38.353, 1.5, 23.5) (38.353, 1.5, 21.5) (38.353, 1.5, 19.5) (38.353, 1.5, 17.5) (38.353, 1.5, 15.5) (38.353, 1.5, 13.5) (38.353, 1.5, 11.5) (38.353, 1.5, 9.5) (38.353, 1.5, 7.5) (38.353, 1.5, 5.5) (38.353, 1.5, 3.5) (38.353, 1.5, 1.5) (40.353, 1.5, 67.5) (40.353, 1.5, 65.5) (40.353, 1.5, 63.5) (40.353, 1.5, 61.5) (40.353, 1.5, 59.5) (40.353, 1.5, 57.5) (40.353, 1.5, 55.5) (40.353, 1.5, 53.5) (40.353, 1.5, 51.5) (40.353, 1.5, 49.5) (40.353, 1.5, 47.5) (40.353, 1.5, 45.5) (40.353, 1.5, 43.5) (40.353, 1.5, 41.5) (40.353, 1.5, 39.5) (40.353, 1.5, 37.5) (40.353, 1.5, 35.5) (40.353, 1.5, 33.5) (40.353, 1.5, 31.5) (40.353, 1.5, 29.5) (40.353, 1.5, 27.5) (40.353, 1.5, 25.5) (40.353, 1.5, 23.5) (40.353, 1.5, 21.5) (40.353, 1.5, 19.5) (40.353, 1.5, 17.5) (40.353, 1.5, 15.5) (40.353, 1.5, 13.5) (40.353, 1.5, 11.5) (40.353, 1.5, 9.5) (40.353, 1.5, 7.5) (40.353, 1.5, 5.5) (40.353, 1.5, 3.5) (40.353, 1.5, 1.5) (42.353, 1.5, 67.5) (42.353, 1.5, 65.5) (42.353, 1.5, 63.5) (42.353, 1.5, 61.5) (42.353, 1.5, 59.5) (42.353, 1.5, 57.5) (42.353, 1.5, 55.5) (42.353, 1.5, 53.5) (42.353, 1.5, 51.5) (42.353, 1.5, 49.5) (42.353, 1.5, 47.5) (42.353, 1.5, 45.5) (42.353, 1.5, 43.5) (42.353, 1.5, 41.5) (42.353, 1.5, 39.5) (42.353, 1.5, 37.5) (42.353, 1.5, 35.5) (42.353, 1.5, 33.5) (42.353, 1.5, 31.5) (42.353, 1.5, 29.5) (42.353, 1.5, 27.5) (42.353, 1.5, 25.5) (42.353, 1.5, 23.5) (42.353, 1.5, 21.5) (42.353, 1.5, 19.5) (42.353, 1.5, 17.5) (42.353, 1.5, 15.5) (42.353, 1.5, 13.5) (42.353, 1.5, 11.5) (42.353, 1.5, 9.5) (42.353, 1.5, 7.5) (42.353, 1.5, 5.5) (42.353, 1.5, 3.5) (42.353, 1.5, 1.5) (44.353, 1.5, 67.5) (44.353, 1.5, 65.5) (44.353, 1.5, 63.5) (44.353, 1.5, 61.5) (44.353, 1.5, 59.5) (44.353, 1.5, 57.5) (44.353, 1.5, 55.5) (44.353, 1.5, 53.5) (44.353, 1.5, 51.5) (44.353, 1.5, 49.5) (44.353, 1.5, 47.5) (44.353, 1.5, 45.5) (44.353, 1.5, 43.5) (44.353, 1.5, 41.5) (44.353, 1.5, 39.5) (44.353, 1.5, 37.5) (44.353, 1.5, 35.5) (44.353, 1.5, 33.5) (44.353, 1.5, 31.5) (44.353, 1.5, 29.5) (44.353, 1.5, 27.5) (44.353, 1.5, 25.5) (44.353, 1.5, 23.5) (44.353, 1.5, 21.5) (44.353, 1.5, 19.5) (44.353, 1.5, 17.5) (44.353, 1.5, 15.5) (44.353, 1.5, 13.5) (44.353, 1.5, 11.5) (44.353, 1.5, 9.5) (44.353, 1.5, 7.5) (44.353, 1.5, 5.5) (44.353, 1.5, 3.5) (44.353, 1.5, 1.5) (46.353, 1.5, 67.5) (46.353, 1.5, 65.5) (46.353, 1.5, 63.5) (46.353, 1.5, 61.5) (46.353, 1.5, 59.5) (46.353, 1.5, 57.5) (46.353, 1.5, 55.5) (46.353, 1.5, 53.5) (46.353, 1.5, 51.5) (46.353, 1.5, 49.5) (46.353, 1.5, 47.5) (46.353, 1.5, 45.5) (46.353, 1.5, 43.5) (46.353, 1.5, 41.5) (46.353, 1.5, 39.5) (46.353, 1.5, 37.5) (46.353, 1.5, 35.5) (46.353, 1.5, 33.5) (46.353, 1.5, 31.5) (46.353, 1.5, 29.5) (46.353, 1.5, 27.5) (46.353, 1.5, 25.5) (46.353, 1.5, 23.5) (46.353, 1.5, 21.5) (46.353, 1.5, 19.5) (46.353, 1.5, 17.5) (46.353, 1.5, 15.5) (46.353, 1.5, 13.5) (46.353, 1.5, 11.5) (46.353, 1.5, 9.5) (46.353, 1.5, 7.5) (46.353, 1.5, 5.5) (46.353, 1.5, 3.5) (46.353, 1.5, 1.5) (48.353, 1.5, 67.5) (48.353, 1.5, 65.5) (48.353, 1.5, 63.5) (48.353, 1.5, 61.5) (48.353, 1.5, 59.5) (48.353, 1.5, 57.5) (48.353, 1.5, 55.5) (48.353, 1.5, 53.5) (48.353, 1.5, 51.5) (48.353, 1.5, 49.5) (48.353, 1.5, 47.5) (48.353, 1.5, 45.5) (48.353, 1.5, 43.5) (48.353, 1.5, 41.5) (48.353, 1.5, 39.5) (48.353, 1.5, 37.5) (48.353, 1.5, 35.5) (48.353, 1.5, 33.5) (48.353, 1.5, 31.5) (48.353, 1.5, 29.5) (48.353, 1.5, 27.5) (48.353, 1.5, 25.5) (48.353, 1.5, 23.5) (48.353, 1.5, 21.5) (48.353, 1.5, 19.5) (48.353, 1.5, 17.5) (48.353, 1.5, 15.5) (48.353, 1.5, 13.5) (48.353, 1.5, 11.5) (48.353, 1.5, 9.5) (48.353, 1.5, 7.5) (48.353, 1.5, 5.5) (48.353, 1.5, 3.5) (48.353, 1.5, 1.5) (-23.647, 1.5, 67.5) (-23.647, 1.5, 65.5) (-23.647, 1.5, 63.5) (-23.647, 1.5, 61.5) (-23.647, 1.5, 59.5) (-23.647, 1.5, 57.5) (-23.647, 1.5, 55.5) (-23.647, 1.5, 53.5) (-23.647, 1.5, 51.5) (-23.647, 1.5, 49.5) (-23.647, 1.5, 47.5) (-23.647, 1.5, 45.5) (-23.647, 1.5, 43.5) (-23.647, 1.5, 41.5) (-23.647, 1.5, 39.5) (-23.647, 1.5, 37.5) (-23.647, 1.5, 35.5) (-23.647, 1.5, 33.5) (-23.647, 1.5, 31.5) (-23.647, 1.5, 29.5) (-23.647, 1.5, 27.5) (-23.647, 1.5, 25.5) (-23.647, 1.5, 23.5) (-23.647, 1.5, 21.5) (-23.647, 1.5, 19.5) (-23.647, 1.5, 17.5) (-23.647, 1.5, 15.5) (-23.647, 1.5, 13.5) (-23.647, 1.5, 11.5) (-23.647, 1.5, 9.5) (-23.647, 1.5, 7.5) (-23.647, 1.5, 5.5) (-23.647, 1.5, 3.5) (-23.647, 1.5, 1.5) (-25.647, 1.5, 67.5) (-25.647, 1.5, 65.5) (-25.647, 1.5, 63.5) (-25.647, 1.5, 61.5) (-25.647, 1.5, 59.5) (-25.647, 1.5, 57.5) (-25.647, 1.5, 55.5) (-25.647, 1.5, 53.5) (-25.647, 1.5, 51.5) (-25.647, 1.5, 49.5) (-25.647, 1.5, 47.5) (-25.647, 1.5, 45.5) (-25.647, 1.5, 43.5) (-25.647, 1.5, 41.5) (-25.647, 1.5, 39.5) (-25.647, 1.5, 37.5) (-25.647, 1.5, 35.5) (-25.647, 1.5, 33.5) (-25.647, 1.5, 31.5) (-25.647, 1.5, 29.5) (-25.647, 1.5, 27.5) (-25.647, 1.5, 25.5) (-25.647, 1.5, 23.5) (-25.647, 1.5, 21.5) (-25.647, 1.5, 19.5) (-25.647, 1.5, 17.5) (-25.647, 1.5, 15.5) (-25.647, 1.5, 13.5) (-25.647, 1.5, 11.5) (-25.647, 1.5, 9.5) (-25.647, 1.5, 7.5) (-25.647, 1.5, 5.5) (-25.647, 1.5, 3.5) (-25.647, 1.5, 1.5) (-27.647, 1.5, 67.5) (-27.647, 1.5, 65.5) (-27.647, 1.5, 63.5) (-27.647, 1.5, 61.5) (-27.647, 1.5, 59.5) (-27.647, 1.5, 57.5) (-27.647, 1.5, 55.5) (-27.647, 1.5, 53.5) (-27.647, 1.5, 51.5) (-27.647, 1.5, 49.5) (-27.647, 1.5, 47.5) (-27.647, 1.5, 45.5) (-27.647, 1.5, 43.5) (-27.647, 1.5, 41.5) (-27.647, 1.5, 39.5) (-27.647, 1.5, 37.5) (-27.647, 1.5, 35.5) (-27.647, 1.5, 33.5) (-27.647, 1.5, 31.5) (-27.647, 1.5, 29.5) (-27.647, 1.5, 27.5) (-27.647, 1.5, 25.5) (-27.647, 1.5, 23.5) (-27.647, 1.5, 21.5) (-27.647, 1.5, 19.5) (-27.647, 1.5, 17.5) (-27.647, 1.5, 15.5) (-27.647, 1.5, 13.5) (-27.647, 1.5, 11.5) (-27.647, 1.5, 9.5) (-27.647, 1.5, 7.5) (-27.647, 1.5, 5.5) (-27.647, 1.5, 3.5) (-27.647, 1.5, 1.5) (-29.647, 1.5, 67.5) (-29.647, 1.5, 65.5) (-29.647, 1.5, 63.5) (-29.647, 1.5, 61.5) (-29.647, 1.5, 59.5) (-29.647, 1.5, 57.5) (-29.647, 1.5, 55.5) (-29.647, 1.5, 53.5) (-29.647, 1.5, 51.5) (-29.647, 1.5, 49.5) (-29.647, 1.5, 47.5) (-29.647, 1.5, 45.5) (-29.647, 1.5, 43.5) (-29.647, 1.5, 41.5) (-29.647, 1.5, 39.5) (-29.647, 1.5, 37.5) (-29.647, 1.5, 35.5) (-29.647, 1.5, 33.5) (-29.647, 1.5, 31.5) (-29.647, 1.5, 29.5) (-29.647, 1.5, 27.5) (-29.647, 1.5, 25.5) (-29.647, 1.5, 23.5) (-29.647, 1.5, 21.5) (-29.647, 1.5, 19.5) (-29.647, 1.5, 17.5) (-29.647, 1.5, 15.5) (-29.647, 1.5, 13.5) (-29.647, 1.5, 11.5) (-29.647, 1.5, 9.5) (-29.647, 1.5, 7.5) (-29.647, 1.5, 5.5) (-29.647, 1.5, 3.5) (-29.647, 1.5, 1.5) (-31.647, 1.5, 67.5) (-31.647, 1.5, 65.5) (-31.647, 1.5, 63.5) (-31.647, 1.5, 61.5) (-31.647, 1.5, 59.5) (-31.647, 1.5, 57.5) (-31.647, 1.5, 55.5) (-31.647, 1.5, 53.5) (-31.647, 1.5, 51.5) (-31.647, 1.5, 49.5) (-31.647, 1.5, 47.5) (-31.647, 1.5, 45.5) (-31.647, 1.5, 43.5) (-31.647, 1.5, 41.5) (-31.647, 1.5, 39.5) (-31.647, 1.5, 37.5) (-31.647, 1.5, 35.5) (-31.647, 1.5, 33.5) (-31.647, 1.5, 31.5) (-31.647, 1.5, 29.5) (-31.647, 1.5, 27.5) (-31.647, 1.5, 25.5) (-31.647, 1.5, 23.5) (-31.647, 1.5, 21.5) (-31.647, 1.5, 19.5) (-31.647, 1.5, 17.5) (-31.647, 1.5, 15.5) (-31.647, 1.5, 13.5) (-31.647, 1.5, 11.5) (-31.647, 1.5, 9.5) (-31.647, 1.5, 7.5) (-31.647, 1.5, 5.5) (-31.647, 1.5, 3.5) (-31.647, 1.5, 1.5) (-33.647, 1.5, 67.5) (-33.647, 1.5, 65.5) (-33.647, 1.5, 63.5) (-33.647, 1.5, 61.5) (-33.647, 1.5, 59.5) (-33.647, 1.5, 57.5) (-33.647, 1.5, 55.5) (-33.647, 1.5, 53.5) (-33.647, 1.5, 51.5) (-33.647, 1.5, 49.5) (-33.647, 1.5, 47.5) (-33.647, 1.5, 45.5) (-33.647, 1.5, 43.5) (-33.647, 1.5, 41.5) (-33.647, 1.5, 39.5) (-33.647, 1.5, 37.5) (-33.647, 1.5, 35.5) (-33.647, 1.5, 33.5) (-33.647, 1.5, 31.5) (-33.647, 1.5, 29.5) (-33.647, 1.5, 27.5) (-33.647, 1.5, 25.5) (-33.647, 1.5, 23.5) (-33.647, 1.5, 21.5) (-33.647, 1.5, 19.5) (-33.647, 1.5, 17.5) (-33.647, 1.5, 15.5) (-33.647, 1.5, 13.5) (-33.647, 1.5, 11.5) (-33.647, 1.5, 9.5) (-33.647, 1.5, 7.5) (-33.647, 1.5, 5.5) (-33.647, 1.5, 3.5) (-33.647, 1.5, 1.5) (-35.647, 1.5, 67.5) (-35.647, 1.5, 65.5) (-35.647, 1.5, 63.5) (-35.647, 1.5, 61.5) (-35.647, 1.5, 59.5) (-35.647, 1.5, 57.5) (-35.647, 1.5, 55.5) (-35.647, 1.5, 53.5) (-35.647, 1.5, 51.5) (-35.647, 1.5, 49.5) (-35.647, 1.5, 47.5) (-35.647, 1.5, 45.5) (-35.647, 1.5, 43.5) (-35.647, 1.5, 41.5) (-35.647, 1.5, 39.5) (-35.647, 1.5, 37.5) (-35.647, 1.5, 35.5) (-35.647, 1.5, 33.5) (-35.647, 1.5, 31.5) (-35.647, 1.5, 29.5) (-35.647, 1.5, 27.5) (-35.647, 1.5, 25.5) (-35.647, 1.5, 23.5) (-35.647, 1.5, 21.5) (-35.647, 1.5, 19.5) (-35.647, 1.5, 17.5) (-35.647, 1.5, 15.5) (-35.647, 1.5, 13.5) (-35.647, 1.5, 11.5) (-35.647, 1.5, 9.5) (-35.647, 1.5, 7.5) (-35.647, 1.5, 5.5) (-35.647, 1.5, 3.5) (-35.647, 1.5, 1.5) (-37.647, 1.5, 67.5) (-37.647, 1.5, 65.5) (-37.647, 1.5, 63.5) (-37.647, 1.5, 61.5) (-37.647, 1.5, 59.5) (-37.647, 1.5, 57.5) (-37.647, 1.5, 55.5) (-37.647, 1.5, 53.5) (-37.647, 1.5, 51.5) (-37.647, 1.5, 49.5) (-37.647, 1.5, 47.5) (-37.647, 1.5, 45.5) (-37.647, 1.5, 43.5) (-37.647, 1.5, 41.5) (-37.647, 1.5, 39.5) (-37.647, 1.5, 37.5) (-37.647, 1.5, 35.5) (-37.647, 1.5, 33.5) (-37.647, 1.5, 31.5) (-37.647, 1.5, 29.5) (-37.647, 1.5, 27.5) (-37.647, 1.5, 25.5) (-37.647, 1.5, 23.5) (-37.647, 1.5, 21.5) (-37.647, 1.5, 19.5) (-37.647, 1.5, 17.5) (-37.647, 1.5, 15.5) (-37.647, 1.5, 13.5) (-37.647, 1.5, 11.5) (-37.647, 1.5, 9.5) (-37.647, 1.5, 7.5) (-37.647, 1.5, 5.5) (-37.647, 1.5, 3.5) (-37.647, 1.5, 1.5) (-39.647, 1.5, 67.5) (-39.647, 1.5, 65.5) (-39.647, 1.5, 63.5) (-39.647, 1.5, 61.5) (-39.647, 1.5, 59.5) (-39.647, 1.5, 57.5) (-39.647, 1.5, 55.5) (-39.647, 1.5, 53.5) (-39.647, 1.5, 51.5) (-39.647, 1.5, 49.5) (-39.647, 1.5, 47.5) (-39.647, 1.5, 45.5) (-39.647, 1.5, 43.5) (-39.647, 1.5, 41.5) (-39.647, 1.5, 39.5) (-39.647, 1.5, 37.5) (-39.647, 1.5, 35.5) (-39.647, 1.5, 33.5) (-39.647, 1.5, 31.5) (-39.647, 1.5, 29.5) (-39.647, 1.5, 27.5) (-39.647, 1.5, 25.5) (-39.647, 1.5, 23.5) (-39.647, 1.5, 21.5) (-39.647, 1.5, 19.5) (-39.647, 1.5, 17.5) (-39.647, 1.5, 15.5) (-39.647, 1.5, 13.5) (-39.647, 1.5, 11.5) (-39.647, 1.5, 9.5) (-39.647, 1.5, 7.5) (-39.647, 1.5, 5.5) (-39.647, 1.5, 3.5) (-39.647, 1.5, 1.5) (-41.647, 1.5, 67.5) (-41.647, 1.5, 65.5) (-41.647, 1.5, 63.5) (-41.647, 1.5, 61.5) (-41.647, 1.5, 59.5) (-41.647, 1.5, 57.5) (-41.647, 1.5, 55.5) (-41.647, 1.5, 53.5) (-41.647, 1.5, 51.5) (-41.647, 1.5, 49.5) (-41.647, 1.5, 47.5) (-41.647, 1.5, 45.5) (-41.647, 1.5, 43.5) (-41.647, 1.5, 41.5) (-41.647, 1.5, 39.5) (-41.647, 1.5, 37.5) (-41.647, 1.5, 35.5) (-41.647, 1.5, 33.5) (-41.647, 1.5, 31.5) (-41.647, 1.5, 29.5) (-41.647, 1.5, 27.5) (-41.647, 1.5, 25.5) (-41.647, 1.5, 23.5) (-41.647, 1.5, 21.5) (-41.647, 1.5, 19.5) (-41.647, 1.5, 17.5) (-41.647, 1.5, 15.5) (-41.647, 1.5, 13.5) (-41.647, 1.5, 11.5) (-41.647, 1.5, 9.5) (-41.647, 1.5, 7.5) (-41.647, 1.5, 5.5) (-41.647, 1.5, 3.5) (-41.647, 1.5, 1.5) (-43.647, 1.5, 67.5) (-43.647, 1.5, 65.5) (-43.647, 1.5, 63.5) (-43.647, 1.5, 61.5) (-43.647, 1.5, 59.5) (-43.647, 1.5, 57.5) (-43.647, 1.5, 55.5) (-43.647, 1.5, 53.5) (-43.647, 1.5, 51.5) (-43.647, 1.5, 49.5) (-43.647, 1.5, 47.5) (-43.647, 1.5, 45.5) (-43.647, 1.5, 43.5) (-43.647, 1.5, 41.5) (-43.647, 1.5, 39.5) (-43.647, 1.5, 37.5) (-43.647, 1.5, 35.5) (-43.647, 1.5, 33.5) (-43.647, 1.5, 31.5) (-43.647, 1.5, 29.5) (-43.647, 1.5, 27.5) (-43.647, 1.5, 25.5) (-43.647, 1.5, 23.5) (-43.647, 1.5, 21.5) (-43.647, 1.5, 19.5) (-43.647, 1.5, 17.5) (-43.647, 1.5, 15.5) (-43.647, 1.5, 13.5) (-43.647, 1.5, 11.5) (-43.647, 1.5, 9.5) (-43.647, 1.5, 7.5) (-43.647, 1.5, 5.5) (-43.647, 1.5, 3.5) (-43.647, 1.5, 1.5) (-45.647, 1.5, 67.5) (-45.647, 1.5, 65.5) (-45.647, 1.5, 63.5) (-45.647, 1.5, 61.5) (-45.647, 1.5, 59.5) (-45.647, 1.5, 57.5) (-45.647, 1.5, 55.5) (-45.647, 1.5, 53.5) (-45.647, 1.5, 51.5) (-45.647, 1.5, 49.5) (-45.647, 1.5, 47.5) (-45.647, 1.5, 45.5) (-45.647, 1.5, 43.5) (-45.647, 1.5, 41.5) (-45.647, 1.5, 39.5) (-45.647, 1.5, 37.5) (-45.647, 1.5, 35.5) (-45.647, 1.5, 33.5) (-45.647, 1.5, 31.5) (-45.647, 1.5, 29.5) (-45.647, 1.5, 27.5) (-45.647, 1.5, 25.5) (-45.647, 1.5, 23.5) (-45.647, 1.5, 21.5) (-45.647, 1.5, 19.5) (-45.647, 1.5, 17.5) (-45.647, 1.5, 15.5) (-45.647, 1.5, 13.5) (-45.647, 1.5, 11.5) (-45.647, 1.5, 9.5) (-45.647, 1.5, 7.5) (-45.647, 1.5, 5.5) (-45.647, 1.5, 3.5) (-45.647, 1.5, 1.5) (-47.647, 1.5, 67.5) (-47.647, 1.5, 65.5) (-47.647, 1.5, 63.5) (-47.647, 1.5, 61.5) (-47.647, 1.5, 59.5) (-47.647, 1.5, 57.5) (-47.647, 1.5, 55.5) (-47.647, 1.5, 53.5) (-47.647, 1.5, 51.5) (-47.647, 1.5, 49.5) (-47.647, 1.5, 47.5) (-47.647, 1.5, 45.5) (-47.647, 1.5, 43.5) (-47.647, 1.5, 41.5) (-47.647, 1.5, 39.5) (-47.647, 1.5, 37.5) (-47.647, 1.5, 35.5) (-47.647, 1.5, 33.5) (-47.647, 1.5, 31.5) (-47.647, 1.5, 29.5) (-47.647, 1.5, 27.5) (-47.647, 1.5, 25.5) (-47.647, 1.5, 23.5) (-47.647, 1.5, 21.5) (-47.647, 1.5, 19.5) (-47.647, 1.5, 17.5) (-47.647, 1.5, 15.5) (-47.647, 1.5, 13.5) (-47.647, 1.5, 11.5) (-47.647, 1.5, 9.5) (-47.647, 1.5, 7.5) (-47.647, 1.5, 5.5) (-47.647, 1.5, 3.5) (-47.647, 1.5, 1.5)
sketch "Skizze3" plane through (0, 1.5, 0) normal (0, 1, 0) x (1, 0, 0)
  line L0 (-50.2277, -69) -> (50.2277, -69) projected
  line L1 (-50.2277, -69) -> (50.2277, -69)
  line L2 (50.2277, -69) -> (50.2277, -66.5)
  line L3 (50.2277, -66.5) -> (-50.2277, -66.5)
  line L4 (-50.2277, -66.5) -> (-50.2277, -69)
  point P0 (0, 0)
  dimension "d41" = 2.5
  constraints: 8 end point, 2 parallel, 1 horizontal, 1 perpendicular
  measures "d41" distance between parallel lines of L3 L0
extrude "Extrusion2" cut sketch "Skizze3" against normal blind 10
